Autodesk Inventor part; units mm, degrees
(part 2 of 2)
  arc A586 (72.5833, -71.3455) -> (69.8846, -69.0178) centre (57.5837, -86.0076) ccw projected
  arc A587 (72.1248, -72.4647) -> (72.5833, -71.3455) centre (0.3933, -42.4252) ccw projected
  arc A588 (68.5687, -72.23) -> (72.1248, -72.4647) centre (71.7232, -51.4931) ccw projected
  arc A589 (68.097, -73.2866) -> (68.5687, -72.23) centre (0.3933, -42.4252) ccw projected
  arc A590 (70.6457, -75.7776) -> (68.097, -73.2866) centre (54.7636, -89.4788) ccw projected
  arc A591 (70.1185, -76.8661) -> (70.6457, -75.7776) centre (0.3933, -42.4252) ccw projected
  arc A592 (66.5839, -76.4107) -> (70.1185, -76.8661) centre (71.0214, -55.9101) ccw projected
  arc A593 (66.0474, -77.436) -> (66.5839, -76.4107) centre (0.3933, -42.4252) ccw projected
  arc A594 (68.4363, -80.0806) -> (66.0474, -77.436) centre (51.7331, -92.768) ccw projected
  arc A595 (67.8425, -81.1342) -> (68.4363, -80.0806) centre (0.3933, -42.4252) ccw projected
  arc A596 (64.343, -80.4601) -> (67.8425, -81.1342) centre (70.0464, -60.275) ccw projected
  arc A597 (63.7437, -81.45) -> (64.343, -80.4601) centre (0.3933, -42.4252) ccw projected
  arc A598 (65.9637, -84.238) -> (63.7437, -81.45) centre (48.504, -95.8624) ccw projected
  arc A599 (65.3055, -85.2527) -> (65.9637, -84.238) centre (0.3933, -42.4252) ccw projected
  arc A600 (61.8547, -84.3622) -> (65.3055, -85.2527) centre (68.802, -64.5707) ccw projected
  arc A601 (61.195, -85.313) -> (61.8547, -84.3622) centre (0.3933, -42.4252) ccw projected
  arc A602 (63.2374, -88.2336) -> (61.195, -85.313) centre (45.0888, -98.7501) ccw projected
  arc A603 (62.5174, -89.2054) -> (63.2374, -88.2336) centre (0.3933, -42.4252) ccw projected
  arc A604 (59.1286, -88.1021) -> (62.5174, -89.2054) centre (67.2929, -68.7809) ccw projected
  arc A605 (58.4111, -89.01) -> (59.1286, -88.1021) centre (0.3933, -42.4252) ccw projected
  arc A606 (60.2679, -92.052) -> (58.4111, -89.01) centre (41.5006, -101.4198) ccw projected
  arc A607 (59.4889, -92.9771) -> (60.2679, -92.052) centre (0.3933, -42.4252) ccw projected
  arc A608 (56.1752, -91.6653) -> (59.4889, -92.9771) centre (65.525, -72.889) ccw projected
  arc A609 (55.4027, -92.5269) -> (56.1752, -91.6653) centre (0.3933, -42.4252) ccw projected
  arc A610 (57.0668, -95.6784) -> (55.4027, -92.5269) centre (37.7534, -103.8613) ccw projected
  arc A611 (56.2318, -96.5533) -> (57.0668, -95.6784) centre (0.3933, -42.4252) ccw projected
  arc A612 (53.0061, -95.038) -> (56.2318, -96.5533) centre (63.505, -76.8793) ccw projected
  arc A613 (52.1815, -95.8499) -> (53.0061, -95.038) centre (0.3933, -42.4252) ccw projected
  arc A614 (53.6464, -99.0987) -> (52.1815, -95.8499) centre (33.8617, -106.0651) ccw projected
  arc A615 (52.7586, -99.92) -> (53.6464, -99.0987) centre (0.3933, -42.4252) ccw projected
  arc A616 (49.6334, -98.2072) -> (52.7586, -99.92) centre (61.241, -80.7363) ccw projected
  arc A617 (48.7599, -98.9662) -> (49.6334, -98.2072) centre (0.3933, -42.4252) ccw projected
  arc A618 (50.0201, -102.2998) -> (48.7599, -98.9662) centre (29.8405, -108.0228) ccw projected
  arc A619 (49.0829, -103.0644) -> (50.0201, -102.2998) centre (0.3933, -42.4252) ccw projected
  arc A620 (46.0702, -101.1605) -> (49.0829, -103.0644) centre (58.7415, -84.445) ccw projected
  arc A621 (45.1512, -101.8637) -> (46.0702, -101.1605) centre (0.3933, -42.4252) ccw projected
  arc A622 (46.2017, -105.2693) -> (45.1512, -101.8637) centre (25.7053, -109.7266) ccw projected
  arc A623 (45.2188, -105.9741) -> (46.2017, -105.2693) centre (0.3933, -42.4252) ccw projected
  arc A624 (42.3303, -103.8866) -> (45.2188, -105.9741) centre (56.0162, -87.9912) ccw projected
  arc A625 (41.3694, -104.5313) -> (42.3303, -103.8866) centre (0.3933, -42.4252) ccw projected
  arc A626 (42.2061, -107.9956) -> (41.3694, -104.5313) centre (21.4723, -111.17) ccw projected
  arc A627 (41.1813, -108.6379) -> (42.2061, -107.9956) centre (0.3933, -42.4252) ccw projected
  arc A628 (38.4281, -106.3749) -> (41.1813, -108.6379) centre (53.0758, -91.3612) ccw projected
  arc A629 (37.429, -106.9587) -> (38.4281, -106.3749) centre (0.3933, -42.4252) ccw projected
  arc A630 (38.0487, -110.4682) -> (37.429, -106.9587) centre (17.1577, -112.3475) ccw projected
  arc A631 (36.986, -111.0456) -> (38.0487, -110.4682) centre (0.3933, -42.4252) ccw projected
  arc A632 (34.3788, -108.6158) -> (36.986, -111.0456) centre (49.9316, -94.5417) ccw projected
  arc A633 (33.3453, -109.1363) -> (34.3788, -108.6158) centre (0.3933, -42.4252) ccw projected
  arc A634 (33.7456, -112.6776) -> (33.3453, -109.1363) centre (12.7782, -113.2545) ccw projected
  arc A635 (32.6491, -113.1878) -> (33.7456, -112.6776) centre (0.3933, -42.4252) ccw projected
  arc A636 (30.198, -110.6006) -> (32.6491, -113.1878) centre (46.5957, -97.5207) ccw projected
  arc A637 (29.1342, -111.0559) -> (30.198, -110.6006) centre (0.3933, -42.4252) ccw projected
  arc A638 (29.3136, -114.6152) -> (29.1342, -111.0559) centre (8.3508, -113.8875) ccw projected
  arc A639 (28.1874, -115.0563) -> (29.3136, -114.6152) centre (0.3933, -42.4252) ccw projected
  arc A640 (25.902, -112.3217) -> (28.1874, -115.0563) centre (43.081, -100.2865) ccw projected
  arc A641 (24.8118, -112.71) -> (25.902, -112.3217) centre (0.3933, -42.4252) ccw projected
  arc A642 (24.7696, -116.2736) -> (24.8118, -112.71) centre (3.8926, -114.2439) ccw projected
  arc A643 (23.6182, -116.6437) -> (24.7696, -116.2736) centre (0.3933, -42.4252) ccw projected
  arc A644 (21.5072, -113.7724) -> (23.6182, -116.6437) centre (39.4013, -102.8285) ccw projected
  arc A645 (20.395, -114.0921) -> (21.5072, -113.7724) centre (0.3933, -42.4252) ccw projected
  arc A646 (20.1313, -117.6462) -> (20.395, -114.0921) centre (-0.5791, -114.3226) ccw projected
  arc A647 (18.9591, -117.944) -> (20.1313, -117.6462) centre (0.3933, -42.4252) ccw projected
  arc A648 (17.0307, -114.947) -> (18.9591, -117.944) centre (35.5705, -105.1367) ccw projected
  arc A649 (15.9008, -115.197) -> (17.0307, -114.947) centre (0.3933, -42.4252) ccw projected
  arc A650 (15.4167, -118.7278) -> (15.9008, -115.197) centre (-5.047, -114.123) ccw projected
  arc A651 (14.2282, -118.9522) -> (15.4167, -118.7278) centre (0.3933, -42.4252) ccw projected
  arc A652 (12.4899, -115.8411) -> (14.2282, -118.9522) centre (31.6037, -107.2024) ccw projected
  arc A653 (11.3466, -116.0203) -> (12.4899, -115.8411) centre (0.3933, -42.4252) ccw projected
  arc A654 (10.6439, -119.5142) -> (11.3466, -116.0203) centre (-9.494, -113.6461) ccw projected
  arc A655 (9.4438, -119.6643) -> (10.6439, -119.5142) centre (0.3933, -42.4252) ccw projected
  arc A656 (7.9022, -116.4511) -> (9.4438, -119.6643) centre (27.5162, -109.0174) ccw projected
  arc A657 (6.7501, -116.5589) -> (7.9022, -116.4511) centre (0.3933, -42.4252) ccw projected
  circle A658 centre (0.3933, -42.4252) radius 85.5443 projected
  circle A659 centre (0.3933, -42.4252) radius 82.55 projected
  circle A660 centre (0.3933, -42.4252) radius 81.28
  line L7 (-19.7673, 36.3148) -> (20.5539, 36.3148)
  line L8 (-77.8779, -20.5148) -> (-57.7172, 14.4044)
  line L9 (-57.7172, -99.2548) -> (-77.8779, -64.3356)
  line L10 (20.5539, -121.1652) -> (-19.7673, -121.1652)
  line L11 (78.6644, -64.3356) -> (58.5038, -99.2548)
  line L12 (58.5038, 14.4044) -> (78.6644, -20.5148)
  point P0 (0.3933, 36.3148)
  point P1 (-67.7976, -3.0552)
  point P2 (-67.7976, -81.7952)
  point P3 (0.3933, -121.1652)
  point P4 (68.5841, -81.7952)
  point P5 (68.5841, -3.0552)
  point P6 (78.6644, -20.5148)
  point P7 (58.5038, 14.4044)
  point P8 (-19.7673, -121.1652)
  dimension "d1" = 162.56
  dimension "d2" = 78.74
  dimension "d5" = 360
  constraints: 12 end point, 2 point on circle, 1 centre point, 1 coincident, 1 horizontal, 1 midpoint, 25 other
  measures "d1" diameter of A660
  measures "d2" distance of A660.centre point (0.393, 36.315)
extrude "Extrusion1" add sketch "Sketch2" along normal blind 7.62 contours A0 | L0 A1 | A101 A100 A248 A249 A99 A98 A250 A97 A96 A252 A95 A94 A253 A102 A93 A92 A91 A90 A89 A88 A87 A86 A85 A84 A83 A82 A81 A80 A79 A78 A77 A76 A75 A74 A73 A72 A71 A70 A69 A68 A67 A66 A65 A64 A63 A62 A61 A60 A59 A58 A57 A56 A55 A54 A53 A52 A51 A50 A49 A48 A47 A46 A45 A44 A43 A42 A41 A40 A39 A38 A37 A36 A35 A34 A33 A32 A31 A30 A29 A28 A27 A26 A25 A24 A23 A22 A21 A20 A19 A18 A17 A16 A15 A14 A13 A12 A11 A10 A9 A8 A7 A6 A5 A4 A3 A2 | A248 A247 A246 A245 A244 A243 A242 A241 A240 A239 A238 A237 A236 A235 A234 A233 A232 A231 A230 A229 A228 A227 A226 A225 A224 A223 A222 A221 A220 A219 A218 A217 A216 A215 A214 A213 A212 A211 A210 A209 A208 A207 A206 A205 A204 A203 A202 A201 A200 A199 A198 A197 A196 A195 A194 A193 A192 A191 A190 A189 A188 A187 A186 A185 A184 A183 A182 A181 A180 A179 A178 A177 A176 A175 A174 A173 A172 A171 A170 A169 A168 A167 A166 A165 A164 A163 A162 A161 A160 A159 A158 A157 A156 A155 A154 A153 A152 A151 A150 A149 A148 A147 A146 A145 A144 A143 A142 A141 A140 A139 A138 A137 A136 A135 A134 A133 A132 A131 A130 A129 A128 A127 A126 A125 A124 A123 A122 A121 A120 A119 A118 A117 A116 A115 A114 A113 A112 A111 A110 A109 A108 A107 A106 A105 A104 A103 A102 A94 A253 A252 A96 A251 A250 A98 A249 A100 | A100 A249 A248 | A249 A250 A98 A99 A100 | A98 A250 | A250 A251 A252 A96 A97 A98 | A96 A252 | A252 A253 A94 A95 A96 | A94 A102 A253 | L2 L3 L4 L5 L6 L1 | A255 A256 A257 A258 A259 A260 A261 A262 A263 A264 A265 A266 A267 A268 A269 A270 A271 A272 A273 A274 A275 A276 A277 A278 A279 A280 A281 A282 A283 A284 A285 A286 A287 A288 A289 A290 A291 A292 A293 A294 A295 A296 A297 A298 A299 A300 A301 A302 A303 A304 A305 A306 A307 A308 A309 A310 A311 A312 A313 A314 A315 A316 A317 A318 A319 A320 A321 A322 A323 A324 A325 A326 A327 A328 A329 A330 A331 A332 A333 A334 A335 A336 A337 A338 A339 A340 A341 A342 A343 A344 A345 A346 A347 A348 A349 A350 A351 A352 A353 A354 A355 A356 A357 A358 A359 A360 A361 A362 A363 A364 A365 A366 A367 A368 A369 A370 A371 A372 A373 A374 A375 A376 A377 A378 A379 A380 A381 A382 A383 A384 A385 A386 A387 A388 A389 A390 A391 A392 A393 A394 A395 A396 A397 A398 A399 A400 A401 A402 A403 A404 A405 A406 A407 A408 A409 A410 A411 A412 A413 A414 A415 A416 A417 A418 A419 A420 A421 A422 A423 A424 A425 A426 A427 A428 A429 A430 A431 A432 A433 A434 A435 A436 A437 A438 A439 A440 A441 A442 A443 A444 A445 A446 A447 A448 A449 A450 A451 A452 A453 A454 A455 A456 A457 A458 A459 A460 A461 A462 A463 A464 A465 A466 A467 A468 A469 A470 A471 A472 A473 A474 A475 A476 A477 A478 A479 A480 A481 A482 A483 A484 A485 A486 A487 A488 A489 A490 A491 A492 A493 A494 A495 A496 A497 A498 A499 A500 A501 A502 A503 A504 A505 A506 A507 A508 A509 A510 A511 A512 A513 A514 A515 A516 A517 A518 A519 A520 A521 A522 A523 A524 A525 A526 A527 A528 A529 A530 A531 A532 A533 A534 A535 A536 A537 A538 A539 A540 A541 A542 A543 A544 A545 A546 A547 A548 A549 A550 A551 A552 A553 A554 A555 A556 A557 A558 A559 A560 A561 A562 A563 A564 A565 A566 A567 A568 A569 A570 A571 A572 A573 A574 A575 A576 A577 A578 A579 A580 A581 A582 A583 A584 A585 A586 A587 A588 A589 A590 A591 A592 A593 A594 A595 A596 A597 A598 A599 A600 A601 A602 A603 A604 A605 A606 A607 A608 A609 A610 A611 A612 A613 A614 A615 A616 A617 A618 A619 A620 A621 A622 A623 A624 A625 A626 A627 A628 A629 A630 A631 A632 A633 A634 A635 A636 A637 A638 A639 A640 A641 A642 A643 A644 A645 A646 A647 A648 A649 A650 A651 A652 A653 A654 A655 A656 A657 A254 | A660 L11 L10 L9 L8 L7 L12
sketch "Sketch3" plane through (-0.3933, 42.4252, 8.89) normal (0, 0, 1) x (1, 0, 0)
  line L0 (3.5268, 9.2654) -> (-1.9537, 9.7195)
  line L1 (-1.9537, 9.7195) -> (-5.0872, 5.2004)
  line L2 (-5.0872, 5.2004) -> (-2.7402, 0.2271)
  line L3 (-2.7402, 0.2271) -> (2.7402, -0.2271)
  line L4 (2.7402, -0.2271) -> (5.8738, 4.2921)
  line L5 (5.8738, 4.2921) -> (3.5268, 9.2654)
  arc A0 (3.4869, -25.0828) -> (4.2324, -21.6038) centre (-12.0318, -19.9381) ccw
  arc A1 (2.2516, -25.1852) -> (3.4869, -25.0828) centre (0.3933, 4.7462) ccw
  arc A2 (0.9436, -21.8763) -> (2.2516, -25.1852) centre (16.7118, -17.5564) ccw
  arc A3 (-0.157, -21.8763) -> (0.9436, -21.8763) centre (0.3933, 4.7462) ccw
  arc A4 (-1.465, -25.1852) -> (-0.157, -21.8763) centre (-15.9252, -17.5564) ccw
  arc A5 (-2.7003, -25.0828) -> (-1.465, -25.1852) centre (0.3933, 4.7462) ccw
  arc A6 (-3.4458, -21.6038) -> (-2.7003, -25.0828) centre (12.8183, -19.9381) ccw
  arc A7 (-4.5315, -21.4226) -> (-3.4458, -21.6038) centre (0.3933, 4.7462) ccw
  arc A8 (-6.3662, -24.4711) -> (-4.5315, -21.4226) centre (-19.3735, -14.5662) ccw
  arc A9 (-7.5678, -24.1668) -> (-6.3662, -24.4711) centre (0.3933, 4.7462) ccw
  arc A10 (-7.7305, -20.6125) -> (-7.5678, -24.1668) centre (8.586, -21.6465) ccw
  arc A11 (-8.7715, -20.2551) -> (-7.7305, -20.6125) centre (0.3933, 4.7462) ccw
  arc A12 (-11.083, -22.9601) -> (-8.7715, -20.2551) centre (-22.2827, -11.0493) ccw
  arc A13 (-12.2182, -22.4621) -> (-11.083, -22.9601) centre (0.3933, 4.7462) ccw
  arc A14 (-11.7936, -18.9295) -> (-12.2182, -22.4621) centre (4.1301, -22.6351) ccw
  arc A15 (-12.7616, -18.4057) -> (-11.7936, -18.9295) centre (0.3933, 4.7462) ccw
  arc A16 (-15.4868, -20.6932) -> (-12.7616, -18.4057) centre (-24.5733, -7.1016) ccw
  arc A17 (-16.5245, -20.0153) -> (-15.4868, -20.6932) centre (0.3933, 4.7462) ccw
  arc A18 (-15.5243, -16.6007) -> (-16.5245, -20.0153) centre (-0.4277, -22.8767) ccw
  arc A19 (-16.3929, -15.9247) -> (-15.5243, -16.6007) centre (0.3933, 4.7462) ccw
  arc A20 (-19.4574, -17.7325) -> (-16.3929, -15.9247) centre (-26.1828, -2.8306) ccw
  arc A21 (-20.3694, -16.893) -> (-19.4574, -17.7325) centre (0.3933, 4.7462) ccw
  arc A22 (-18.8208, -13.6896) -> (-20.3694, -16.893) centre (-4.963, -22.3648) ccw
  arc A23 (-19.5663, -12.8798) -> (-18.8208, -13.6896) centre (0.3933, 4.7462) ccw
  arc A24 (-22.8866, -14.1586) -> (-19.5663, -12.8798) centre (-27.0675, 1.647) ccw
  arc A25 (-23.6479, -13.1804) -> (-22.8866, -14.1586) centre (0.3933, 4.7462) ccw
  arc A26 (-21.5932, -10.2756) -> (-23.6479, -13.1804) centre (-9.3523, -21.1134) ccw
  arc A27 (-22.1952, -9.3542) -> (-21.5932, -10.2756) centre (0.3933, 4.7462) ccw
  arc A28 (-25.6807, -10.069) -> (-22.1952, -9.3542) centre (-27.2031, 6.2092) ccw
  arc A29 (-26.2707, -8.9789) -> (-25.6807, -10.069) centre (0.3933, 4.7462) ccw
  arc A30 (-23.7659, -6.4519) -> (-26.2707, -8.9789) centre (-13.4758, -19.1567) ccw
  arc A31 (-24.208, -5.4439) -> (-23.7659, -6.4519) centre (0.3933, 4.7462) ccw
  arc A32 (-27.7636, -5.5753) -> (-24.208, -5.4439) centre (-26.5859, 10.7314) ccw
  arc A33 (-28.1661, -4.4029) -> (-27.7636, -5.5753) centre (0.3933, 4.7462) ccw
  arc A34 (-25.2795, -2.3227) -> (-28.1661, -4.4029) centre (-17.2209, -16.5479) ccw
  arc A35 (-25.5497, -1.2557) -> (-25.2795, -2.3227) centre (0.3933, 4.7462) ccw
  arc A36 (-29.0784, -0.8001) -> (-25.5497, -1.2557) centre (-25.2328, 15.0904) ccw
  arc A37 (-29.2825, 0.4226) -> (-29.0784, -0.8001) centre (0.3933, 4.7462) ccw
  arc A38 (-26.0929, 1.9993) -> (-29.2825, 0.4226) centre (-20.4856, -13.3583) ccw
  arc A39 (-26.1838, 3.0962) -> (-26.0929, 1.9993) centre (0.3933, 4.7462) ccw
  arc A40 (-29.5894, 4.1265) -> (-26.1838, 3.0962) centre (-23.1807, 19.1673) ccw
  arc A41 (-29.5894, 5.366) -> (-29.5894, 4.1265) centre (0.3933, 4.7462) ccw
  arc A42 (-26.1838, 6.3963) -> (-29.5894, 5.366) centre (-23.1807, -9.6748) ccw
  arc A43 (-26.0929, 7.4931) -> (-26.1838, 6.3963) centre (0.3933, 4.7462) ccw
  arc A44 (-29.2825, 9.0699) -> (-26.0929, 7.4931) centre (-20.4856, 22.8507) ccw
  arc A45 (-29.0784, 10.2925) -> (-29.2825, 9.0699) centre (0.3933, 4.7462) ccw
  arc A46 (-25.5497, 10.7482) -> (-29.0784, 10.2925) centre (-25.2328, -5.598) ccw
  arc A47 (-25.2795, 11.8152) -> (-25.5497, 10.7482) centre (0.3933, 4.7462) ccw
  arc A48 (-28.1661, 13.8954) -> (-25.2795, 11.8152) centre (-17.2209, 26.0404) ccw
  arc A49 (-27.7636, 15.0678) -> (-28.1661, 13.8954) centre (0.3933, 4.7462) ccw
  arc A50 (-24.208, 14.9364) -> (-27.7636, 15.0678) centre (-26.5859, -1.239) ccw
  arc A51 (-23.7659, 15.9444) -> (-24.208, 14.9364) centre (0.3933, 4.7462) ccw
  arc A52 (-26.2707, 18.4713) -> (-23.7659, 15.9444) centre (-13.4758, 28.6491) ccw
  arc A53 (-25.6807, 19.5615) -> (-26.2707, 18.4713) centre (0.3933, 4.7462) ccw
  arc A54 (-22.1952, 18.8467) -> (-25.6807, 19.5615) centre (-27.2031, 3.2833) ccw
  arc A55 (-21.5932, 19.7681) -> (-22.1952, 18.8467) centre (0.3933, 4.7462) ccw
  arc A56 (-23.6479, 22.6729) -> (-21.5932, 19.7681) centre (-9.3523, 30.6059) ccw
  arc A57 (-22.8866, 23.6511) -> (-23.6479, 22.6729) centre (0.3933, 4.7462) ccw
  arc A58 (-19.5663, 22.3723) -> (-22.8866, 23.6511) centre (-27.0675, 7.8455) ccw
  arc A59 (-18.8208, 23.1821) -> (-19.5663, 22.3723) centre (0.3933, 4.7462) ccw
  arc A60 (-20.3694, 26.3854) -> (-18.8208, 23.1821) centre (-4.963, 31.8573) ccw
  arc A61 (-19.4574, 27.225) -> (-20.3694, 26.3854) centre (0.3933, 4.7462) ccw
  arc A62 (-16.3929, 25.4171) -> (-19.4574, 27.225) centre (-26.1828, 12.3231) ccw
  arc A63 (-15.5243, 26.0932) -> (-16.3929, 25.4171) centre (0.3933, 4.7462) ccw
  arc A64 (-16.5245, 29.5077) -> (-15.5243, 26.0932) centre (-0.4277, 32.3691) ccw
  arc A65 (-15.4868, 30.1857) -> (-16.5245, 29.5077) centre (0.3933, 4.7462) ccw
  arc A66 (-12.7616, 27.8981) -> (-15.4868, 30.1857) centre (-24.5733, 16.594) ccw
  arc A67 (-11.7936, 28.422) -> (-12.7616, 27.8981) centre (0.3933, 4.7462) ccw
  arc A68 (-12.2182, 31.9546) -> (-11.7936, 28.422) centre (4.1301, 32.1275) ccw
  arc A69 (-11.083, 32.4525) -> (-12.2182, 31.9546) centre (0.3933, 4.7462) ccw
  arc A70 (-8.7715, 29.7476) -> (-11.083, 32.4525) centre (-22.2827, 20.5418) ccw
  arc A71 (-7.7305, 30.105) -> (-8.7715, 29.7476) centre (0.3933, 4.7462) ccw
  arc A72 (-7.5678, 33.6593) -> (-7.7305, 30.105) centre (8.586, 31.139) ccw
  arc A73 (-6.3662, 33.9636) -> (-7.5678, 33.6593) centre (0.3933, 4.7462) ccw
  arc A74 (-4.5315, 30.9151) -> (-6.3662, 33.9636) centre (-19.3735, 24.0587) ccw
  arc A75 (-3.4458, 31.0962) -> (-4.5315, 30.9151) centre (0.3933, 4.7462) ccw
  arc A76 (-2.7003, 34.5753) -> (-3.4458, 31.0962) centre (12.8183, 29.4306) ccw
  arc A77 (-1.465, 34.6777) -> (-2.7003, 34.5753) centre (0.3933, 4.7462) ccw
  arc A78 (-0.157, 31.3688) -> (-1.465, 34.6777) centre (-15.9252, 27.0488) ccw
  arc A79 (0.9436, 31.3688) -> (-0.157, 31.3688) centre (0.3933, 4.7462) ccw
  arc A80 (2.2516, 34.6777) -> (0.9436, 31.3688) centre (16.7118, 27.0488) ccw
  arc A81 (3.4869, 34.5753) -> (2.2516, 34.6777) centre (0.3933, 4.7462) ccw
  arc A82 (4.2324, 31.0962) -> (3.4869, 34.5753) centre (-12.0318, 29.4306) ccw
  arc A83 (5.318, 30.9151) -> (4.2324, 31.0962) centre (0.3933, 4.7462) ccw
  arc A84 (7.1528, 33.9636) -> (5.318, 30.9151) centre (20.1601, 24.0587) ccw
  arc A85 (8.3544, 33.6593) -> (7.1528, 33.9636) centre (0.3933, 4.7462) ccw
  arc A86 (8.5171, 30.105) -> (8.3544, 33.6593) centre (-7.7994, 31.139) ccw
  arc A87 (9.5581, 29.7476) -> (8.5171, 30.105) centre (0.3933, 4.7462) ccw
  arc A88 (11.8696, 32.4525) -> (9.5581, 29.7476) centre (23.0692, 20.5418) ccw
  arc A89 (13.0048, 31.9546) -> (11.8696, 32.4525) centre (0.3933, 4.7462) ccw
  arc A90 (12.5802, 28.422) -> (13.0048, 31.9546) centre (-3.3436, 32.1275) ccw
  arc A91 (13.5482, 27.8981) -> (12.5802, 28.422) centre (0.3933, 4.7462) ccw
  arc A92 (16.2734, 30.1857) -> (13.5482, 27.8981) centre (25.3598, 16.594) ccw
  arc A93 (17.3111, 29.5077) -> (16.2734, 30.1857) centre (0.3933, 4.7462) ccw
  arc A94 (16.3109, 26.0932) -> (17.3111, 29.5077) centre (1.2142, 32.3691) ccw
  arc A95 (17.1795, 25.4171) -> (16.3109, 26.0932) centre (0.3933, 4.7462) ccw
  arc A96 (20.244, 27.225) -> (17.1795, 25.4171) centre (26.9694, 12.3231) ccw
  arc A97 (21.156, 26.3854) -> (20.244, 27.225) centre (0.3933, 4.7462) ccw
  arc A98 (19.6074, 23.1821) -> (21.156, 26.3854) centre (5.7496, 31.8573) ccw
  arc A99 (20.3528, 22.3723) -> (19.6074, 23.1821) centre (0.3933, 4.7462) ccw
  arc A100 (23.6731, 23.6511) -> (20.3528, 22.3723) centre (27.854, 7.8455) ccw
  arc A101 (24.4345, 22.6729) -> (23.6731, 23.6511) centre (0.3933, 4.7462) ccw
  arc A102 (22.3798, 19.7681) -> (24.4345, 22.6729) centre (10.1389, 30.6059) ccw
  arc A103 (22.9818, 18.8467) -> (22.3798, 19.7681) centre (0.3933, 4.7462) ccw
  arc A104 (26.4673, 19.5615) -> (22.9818, 18.8467) centre (27.9896, 3.2833) ccw
  arc A105 (27.0572, 18.4713) -> (26.4673, 19.5615) centre (0.3933, 4.7462) ccw
  arc A106 (24.5524, 15.9444) -> (27.0572, 18.4713) centre (14.2623, 28.6491) ccw
  arc A107 (24.9945, 14.9364) -> (24.5524, 15.9444) centre (0.3933, 4.7462) ccw
  arc A108 (28.5502, 15.0678) -> (24.9945, 14.9364) centre (27.3725, -1.239) ccw
  arc A109 (28.9527, 13.8954) -> (28.5502, 15.0678) centre (0.3933, 4.7462) ccw
  arc A110 (26.0661, 11.8152) -> (28.9527, 13.8954) centre (18.0075, 26.0404) ccw
  arc A111 (26.3363, 10.7482) -> (26.0661, 11.8152) centre (0.3933, 4.7462) ccw
  arc A112 (29.865, 10.2925) -> (26.3363, 10.7482) centre (26.0194, -5.598) ccw
  arc A113 (30.069, 9.0699) -> (29.865, 10.2925) centre (0.3933, 4.7462) ccw
  arc A114 (26.8794, 7.4931) -> (30.069, 9.0699) centre (21.2721, 22.8507) ccw
  arc A115 (26.9703, 6.3963) -> (26.8794, 7.4931) centre (0.3933, 4.7462) ccw
  arc A116 (30.376, 5.366) -> (26.9703, 6.3963) centre (23.9673, -9.6748) ccw
  arc A117 (30.376, 4.1265) -> (30.376, 5.366) centre (0.3933, 4.7462) ccw
  arc A118 (26.9703, 3.0962) -> (30.376, 4.1265) centre (23.9673, 19.1673) ccw
  arc A119 (26.8794, 1.9993) -> (26.9703, 3.0962) centre (0.3933, 4.7462) ccw
  arc A120 (30.069, 0.4226) -> (26.8794, 1.9993) centre (21.2721, -13.3583) ccw
  arc A121 (29.865, -0.8001) -> (30.069, 0.4226) centre (0.3933, 4.7462) ccw
  arc A122 (26.3363, -1.2557) -> (29.865, -0.8001) centre (26.0194, 15.0904) ccw
  arc A123 (26.0661, -2.3227) -> (26.3363, -1.2557) centre (0.3933, 4.7462) ccw
  arc A124 (28.9527, -4.4029) -> (26.0661, -2.3227) centre (18.0075, -16.5479) ccw
  arc A125 (28.5502, -5.5753) -> (28.9527, -4.4029) centre (0.3933, 4.7462) ccw
  arc A126 (24.9945, -5.4439) -> (28.5502, -5.5753) centre (27.3725, 10.7314) ccw
  arc A127 (24.5524, -6.4519) -> (24.9945, -5.4439) centre (0.3933, 4.7462) ccw
  arc A128 (27.0572, -8.9789) -> (24.5524, -6.4519) centre (14.2623, -19.1567) ccw
  arc A129 (26.4673, -10.069) -> (27.0572, -8.9789) centre (0.3933, 4.7462) ccw
  arc A130 (22.9818, -9.3542) -> (26.4673, -10.069) centre (27.9896, 6.2092) ccw
  arc A131 (22.3798, -10.2756) -> (22.9818, -9.3542) centre (0.3933, 4.7462) ccw
  arc A132 (24.4345, -13.1804) -> (22.3798, -10.2756) centre (10.1389, -21.1134) ccw
  arc A133 (23.6731, -14.1586) -> (24.4345, -13.1804) centre (0.3933, 4.7462) ccw
  arc A134 (20.3528, -12.8798) -> (23.6731, -14.1586) centre (27.854, 1.647) ccw
  arc A135 (19.6074, -13.6896) -> (20.3528, -12.8798) centre (0.3933, 4.7462) ccw
  arc A136 (21.156, -16.893) -> (19.6074, -13.6896) centre (5.7496, -22.3648) ccw
  arc A137 (20.244, -17.7325) -> (21.156, -16.893) centre (0.3933, 4.7462) ccw
  arc A138 (17.1795, -15.9247) -> (20.244, -17.7325) centre (26.9694, -2.8306) ccw
  arc A139 (16.3109, -16.6007) -> (17.1795, -15.9247) centre (0.3933, 4.7462) ccw
  arc A140 (17.3111, -20.0153) -> (16.3109, -16.6007) centre (1.2142, -22.8767) ccw
  arc A141 (16.2734, -20.6932) -> (17.3111, -20.0153) centre (0.3933, 4.7462) ccw
  arc A142 (13.5482, -18.4057) -> (16.2734, -20.6932) centre (25.3598, -7.1016) ccw
  arc A143 (12.5802, -18.9295) -> (13.5482, -18.4057) centre (0.3933, 4.7462) ccw
  arc A144 (13.0048, -22.4621) -> (12.5802, -18.9295) centre (-3.3436, -22.6351) ccw
  arc A145 (11.8696, -22.9601) -> (13.0048, -22.4621) centre (0.3933, 4.7462) ccw
  arc A146 (9.5581, -20.2551) -> (11.8696, -22.9601) centre (23.0692, -11.0493) ccw
  arc A147 (8.5171, -20.6125) -> (9.5581, -20.2551) centre (0.3933, 4.7462) ccw
  arc A148 (8.3544, -24.1668) -> (8.5171, -20.6125) centre (-7.7994, -21.6465) ccw
  arc A149 (7.1528, -24.4711) -> (8.3544, -24.1668) centre (0.3933, 4.7462) ccw
  arc A150 (5.318, -21.4226) -> (7.1528, -24.4711) centre (20.1601, -14.5662) ccw
  arc A151 (4.2324, -21.6038) -> (5.318, -21.4226) centre (0.3933, 4.7462) ccw
  circle A152 centre (0.3933, 4.7462) radius 14.605
  point P0 (0.3933, -42.4252)
extrude "Extrusion2" cut sketch "Sketch3" against normal through all contours L5 L4 L3 L2 L1 L0 | A152
chamfer "Chamfer1" distance 1 angle 45 1 edges at (-14.605, 47.1714, 8.89)
pattern_circular "Circular Pattern1" count 3 over 360 about axis through (0, 0, 1.27) along (0, 0, 1) of "Extrusion2", "Chamfer1"
sketch "Sketch4" plane through (-0.3933, 42.4252, 8.89) normal (0, 0, 1) x (1, 0, 0)
  arc A0 (0.495, -45.4235) -> (0.2916, -45.4235) centre (0.3933, -42.4252) ccw projected
  line L0 (0.2916, -45.4235) -> (0.495, -45.4235) projected
  arc A1 (-5.2339, -23.0564) -> (-5.3005, -26.6101) centre (8.4164, -25.0898) ccw projected
  arc A2 (-5.3005, -26.6101) -> (-6.2823, -26.9988) centre (0.3933, -42.4252) ccw projected
  arc A3 (-6.2823, -26.9988) -> (-8.7636, -24.4539) centre (-17.3222, -35.2804) ccw projected
  arc A4 (-8.7636, -24.4539) -> (-9.8739, -25.0643) centre (0.3933, -42.4252) ccw projected
  arc A5 (-9.8739, -25.0643) -> (-9.0547, -28.5229) centre (3.8531, -23.6391) ccw projected
  arc A6 (-9.0547, -28.5229) -> (-9.909, -29.1436) centre (0.3933, -42.4252) ccw projected
  arc A7 (-9.909, -29.1436) -> (-12.9452, -27.2957) centre (-18.5425, -39.9105) ccw projected
  arc A8 (-12.9452, -27.2957) -> (-13.8688, -28.1631) centre (0.3933, -42.4252) ccw projected
  arc A9 (-13.8688, -28.1631) -> (-12.2152, -31.3093) centre (-0.9275, -23.3689) ccw projected
  arc A10 (-12.2152, -31.3093) -> (-12.8883, -32.1229) centre (0.3933, -42.4252) ccw projected
  arc A11 (-12.8883, -32.1229) -> (-16.2887, -31.0882) centre (-18.5729, -44.6986) ccw projected
  arc A12 (-16.2887, -31.0882) -> (-16.9676, -32.158) centre (0.3933, -42.4252) ccw projected
  arc A13 (-16.9676, -32.158) -> (-14.5835, -34.7941) centre (-5.6251, -24.296) ccw projected
  arc A14 (-14.5835, -34.7941) -> (-15.0331, -35.7496) centre (0.3933, -42.4252) ccw projected
  arc A15 (-15.0331, -35.7496) -> (-18.584, -35.593) centre (-17.4117, -49.3439) ccw projected
  arc A16 (-18.584, -35.593) -> (-18.9755, -36.798) centre (0.3933, -42.4252) ccw projected
  arc A17 (-18.9755, -36.798) -> (-16.0107, -38.7585) centre (-9.9445, -26.3623) ccw projected
  arc A18 (-16.0107, -38.7585) -> (-16.2086, -39.7957) centre (0.3933, -42.4252) ccw projected
  arc A19 (-16.2086, -39.7957) -> (-19.6869, -40.5271) centre (-15.1317, -53.5545) ccw projected
  arc A20 (-19.6869, -40.5271) -> (-19.7664, -41.7916) centre (0.3933, -42.4252) ccw projected
  arc A21 (-19.7664, -41.7916) -> (-16.4072, -42.9532) centre (-13.6144, -29.4379) ccw projected
  arc A22 (-16.4072, -42.9532) -> (-16.3409, -44.007) centre (0.3933, -42.4252) ccw projected
  arc A23 (-16.3409, -44.007) -> (-19.5281, -45.5804) centre (-11.8762, -57.0657) ccw projected
  arc A24 (-19.5281, -45.5804) -> (-19.2906, -46.8251) centre (0.3933, -42.4252) ccw projected
  arc A25 (-19.2906, -46.8251) -> (-15.7481, -47.1147) centre (-16.4042, -33.3295) ccw projected
  arc A26 (-15.7481, -47.1147) -> (-15.4218, -48.119) centre (0.3933, -42.4252) ccw projected
  arc A27 (-15.4218, -48.119) -> (-18.1175, -50.4355) centre (-7.8498, -59.6571) ccw projected
  arc A28 (-18.1175, -50.4355) -> (-17.578, -51.582) centre (0.3933, -42.4252) ccw projected
  arc A29 (-17.578, -51.582) -> (-14.0748, -50.9816) centre (-18.1385, -37.7926) ccw projected
  arc A30 (-14.0748, -50.9816) -> (-13.509, -51.8732) centre (0.3933, -42.4252) ccw projected
  arc A31 (-13.509, -51.8732) -> (-15.5439, -54.7873) centre (-3.3054, -61.1657) ccw projected
  arc A32 (-15.5439, -54.7873) -> (-14.7362, -55.7636) centre (0.3933, -42.4252) ccw projected
  arc A33 (-14.7362, -55.7636) -> (-11.4923, -54.3108) centre (-18.7083, -42.5468) ccw projected
  arc A34 (-11.4923, -54.3108) -> (-10.7226, -55.0337) centre (0.3933, -42.4252) ccw projected
  arc A35 (-10.7226, -55.0337) -> (-11.9689, -58.3624) centre (1.4713, -61.4968) ccw projected
  arc A36 (-11.9689, -58.3624) -> (-10.9438, -59.1071) centre (0.3933, -42.4252) ccw projected
  arc A37 (-10.9438, -59.1071) -> (-8.1631, -56.8933) centre (-18.078, -47.2933) ccw projected
  arc A38 (-8.1631, -56.8933) -> (-7.2378, -57.402) centre (0.3933, -42.4252) ccw projected
  arc A39 (-7.2378, -57.402) -> (-7.6171, -60.936) centre (6.1804, -60.6295) ccw projected
  arc A40 (-7.6171, -60.936) -> (-6.439, -61.4025) centre (0.3933, -42.4252) ccw projected
  arc A41 (-6.439, -61.4025) -> (-4.2962, -58.5666) centre (-16.287, -51.734) ccw projected
  arc A42 (-4.2962, -58.5666) -> (-3.2734, -58.8292) centre (0.3933, -42.4252) ccw projected
  arc A43 (-3.2734, -58.8292) -> (-2.7619, -62.3466) centre (10.5258, -58.6184) ccw projected
  arc A44 (-2.7619, -62.3466) -> (-1.5049, -62.5054) centre (0.3933, -42.4252) ccw projected
  arc A45 (-1.5049, -62.5054) -> (-0.1347, -59.2257) centre (-13.448, -55.5898) ccw projected
  arc A46 (-0.1347, -59.2257) -> (0.9213, -59.2257) centre (0.3933, -42.4252) ccw projected
  arc A47 (0.9213, -59.2257) -> (2.2914, -62.5054) centre (14.2345, -55.5898) ccw projected
  arc A48 (2.2914, -62.5054) -> (3.5485, -62.3466) centre (0.3933, -42.4252) ccw projected
  arc A49 (3.5485, -62.3466) -> (4.06, -58.8292) centre (-9.7392, -58.6184) ccw projected
  arc A50 (4.06, -58.8292) -> (5.0828, -58.5666) centre (0.3933, -42.4252) ccw projected
  arc A51 (5.0828, -58.5666) -> (7.2255, -61.4025) centre (17.0736, -51.734) ccw projected
  arc A52 (7.2255, -61.4025) -> (8.4036, -60.936) centre (0.3933, -42.4252) ccw projected
  arc A53 (8.4036, -60.936) -> (8.0243, -57.402) centre (-5.3938, -60.6295) ccw projected
  arc A54 (8.0243, -57.402) -> (8.9497, -56.8933) centre (0.3933, -42.4252) ccw projected
  arc A55 (8.9497, -56.8933) -> (11.7303, -59.1071) centre (18.8646, -47.2933) ccw projected
  arc A56 (11.7303, -59.1071) -> (12.7554, -58.3624) centre (0.3933, -42.4252) ccw projected
  arc A57 (12.7554, -58.3624) -> (11.5092, -55.0337) centre (-0.6848, -61.4968) ccw projected
  arc A58 (11.5092, -55.0337) -> (12.2789, -54.3108) centre (0.3933, -42.4252) ccw projected
  arc A59 (12.2789, -54.3108) -> (15.5228, -55.7636) centre (19.4949, -42.5468) ccw projected
  arc A60 (15.5228, -55.7636) -> (16.3305, -54.7873) centre (0.3933, -42.4252) ccw projected
  arc A61 (16.3305, -54.7873) -> (14.2955, -51.8732) centre (4.092, -61.1657) ccw projected
  arc A62 (14.2955, -51.8732) -> (14.8613, -50.9816) centre (0.3933, -42.4252) ccw projected
  arc A63 (14.8613, -50.9816) -> (18.3646, -51.582) centre (18.925, -37.7926) ccw projected
  arc A64 (18.3646, -51.582) -> (18.9041, -50.4355) centre (0.3933, -42.4252) ccw projected
  arc A65 (18.9041, -50.4355) -> (16.2084, -48.119) centre (8.6364, -59.6571) ccw projected
  arc A66 (16.2084, -48.119) -> (16.5347, -47.1147) centre (0.3933, -42.4252) ccw projected
  arc A67 (16.5347, -47.1147) -> (20.0772, -46.8251) centre (17.1907, -33.3295) ccw projected
  arc A68 (20.0772, -46.8251) -> (20.3146, -45.5804) centre (0.3933, -42.4252) ccw projected
  arc A69 (20.3146, -45.5804) -> (17.1275, -44.007) centre (12.6628, -57.0657) ccw projected
  arc A70 (17.1275, -44.007) -> (17.1938, -42.9532) centre (0.3933, -42.4252) ccw projected
  arc A71 (17.1938, -42.9532) -> (20.553, -41.7916) centre (14.401, -29.4379) ccw projected
  arc A72 (20.553, -41.7916) -> (20.4735, -40.5271) centre (0.3933, -42.4252) ccw projected
  arc A73 (20.4735, -40.5271) -> (16.9952, -39.7957) centre (15.9183, -53.5545) ccw projected
  arc A74 (16.9952, -39.7957) -> (16.7973, -38.7585) centre (0.3933, -42.4252) ccw projected
  arc A75 (16.7973, -38.7585) -> (19.7621, -36.798) centre (10.7311, -26.3623) ccw projected
  arc A76 (19.7621, -36.798) -> (19.3706, -35.593) centre (0.3933, -42.4252) ccw projected
  arc A77 (19.3706, -35.593) -> (15.8197, -35.7496) centre (18.1983, -49.3439) ccw projected
  arc A78 (15.8197, -35.7496) -> (15.3701, -34.7941) centre (0.3933, -42.4252) ccw projected
  arc A79 (15.3701, -34.7941) -> (17.7542, -32.158) centre (6.4116, -24.296) ccw projected
  arc A80 (17.7542, -32.158) -> (17.0752, -31.0882) centre (0.3933, -42.4252) ccw projected
  arc A81 (17.0752, -31.0882) -> (13.6749, -32.1229) centre (19.3595, -44.6986) ccw projected
  arc A82 (13.6749, -32.1229) -> (13.0018, -31.3093) centre (0.3933, -42.4252) ccw projected
  arc A83 (13.0018, -31.3093) -> (14.6554, -28.1631) centre (1.714, -23.3689) ccw projected
  arc A84 (14.6554, -28.1631) -> (13.7317, -27.2957) centre (0.3933, -42.4252) ccw projected
  arc A85 (13.7317, -27.2957) -> (10.6955, -29.1436) centre (19.329, -39.9105) ccw projected
  arc A86 (10.6955, -29.1436) -> (9.8412, -28.5229) centre (0.3933, -42.4252) ccw projected
  arc A87 (9.8412, -28.5229) -> (10.6605, -25.0643) centre (-3.0666, -23.6391) ccw projected
  arc A88 (10.6605, -25.0643) -> (9.5501, -24.4539) centre (0.3933, -42.4252) ccw projected
  arc A89 (9.5501, -24.4539) -> (7.0689, -26.9988) centre (18.1088, -35.2804) ccw projected
  arc A90 (7.0689, -26.9988) -> (6.0871, -26.6101) centre (0.3933, -42.4252) ccw projected
  arc A91 (6.0871, -26.6101) -> (6.0204, -23.0564) centre (-7.6298, -25.0898) ccw projected
  arc A92 (6.0204, -23.0564) -> (4.7932, -22.7413) centre (0.3933, -42.4252) ccw projected
  arc A93 (4.7932, -22.7413) -> (3.0228, -25.8233) centre (15.7754, -31.0992) ccw projected
  arc A94 (3.0228, -25.8233) -> (1.9751, -25.691) centre (0.3933, -42.4252) ccw projected
  arc A95 (1.9751, -25.691) -> (1.0268, -22.2655) centre (-11.6889, -27.6297) ccw projected
  arc A96 (1.0268, -22.2655) -> (-0.2403, -22.2655) centre (0.3933, -42.4252) ccw projected
  arc A97 (-0.2403, -22.2655) -> (-1.1886, -25.691) centre (12.4754, -27.6297) ccw projected
  arc A98 (-1.1886, -25.691) -> (-2.2362, -25.8233) centre (0.3933, -42.4252) ccw projected
  arc A99 (-2.2362, -25.8233) -> (-4.0066, -22.7413) centre (-14.9888, -31.0992) ccw projected
  arc A100 (-4.0066, -22.7413) -> (-5.2339, -23.0564) centre (0.3933, -42.4252) ccw projected
  arc A101 (1.0086, -44.8483) -> (-0.222, -44.8483) centre (0.3933, -42.4252) ccw projected
  line L1 (-15.1067, -57.9252) -> (15.8933, -57.9252) construction
  line L2 (15.8933, -57.9252) -> (15.8933, -26.9252) construction
  line L3 (15.8933, -26.9252) -> (-15.1067, -26.9252) construction
  line L4 (-15.1067, -26.9252) -> (-15.1067, -57.9252) construction
  line L5 (-15.1067, -57.9252) -> (15.8933, -26.9252) construction
  line L6 (15.8933, -57.9252) -> (-15.1067, -26.9252) construction
  circle A102 centre (-15.1067, -26.9252) radius 3.175
  circle A103 centre (15.8933, -26.9252) radius 3.175
  circle A104 centre (15.8933, -57.9252) radius 3.175
  circle A105 centre (-15.1067, -57.9252) radius 3.175
  point P0 (0.3933, -42.4252)
  point P1 (14.1509, -55.271)
  point P2 (12.7402, -58.298)
  point P3 (12.7492, -58.3672)
  point P4 (16.3266, -54.7799)
  point P5 (-15.54, -54.7799)
  point P6 (-11.9626, -58.3672)
  point P7 (-11.9537, -58.298)
  point P8 (-13.3644, -55.271)
  dimension "d18" = 31
  dimension "d19" = 31
  dimension "d20" = 6.35
  dimension "d21" = 6.35
  dimension "d22" = 6.35
  dimension "d23" = 6.35
  constraints: 12 end point, 4 centre point, 4 coincident, 2 midpoint, 2 parallel, 1 horizontal, 1 perpendicular
  measures "d18" distance of L3.end L2.end
  measures "d19" distance of L2.end L1.end
  measures "d20" diameter of A102
  measures "d21" diameter of A103
  measures "d22" diameter of A104
  measures "d23" diameter of A105
extrude "Extrusion3" add sketch "Sketch4" along normal blind 10.16 contours A102 A9 A8 A7 | A7 A8 A9 A102 | A103 A83 A84 A85 | A85 A84 A83 A103 | A105 A33 A32 A31 | A31 A32 A33 A105 A35 A36 | A36 A35 A105 | A104 A56 A57 A59 A60 A61 | A61 A60 A59 A104 | A104 A57 A56
sketch "Sketch6" plane through (-0.3933, 42.4252, 1.27) normal (0, 0, -1) x (-1, 0, 0)
  circle A0 centre (15.1067, -57.9252) radius 3.175 projected
  circle A1 centre (15.1067, -26.9252) radius 3.175 projected
  circle A2 centre (-15.8933, -26.9252) radius 3.175 projected
  circle A3 centre (-15.8933, -57.9252) radius 3.175 projected
  point P0 (-0.3933, -42.4252)
hole "Hole2" at (-15.5, -15.5, 1.27) at (-15.5, 15.5, 1.27) at (15.5, -15.5, 1.27) at (15.5, 15.5, 1.27) direction (0, 0, 1) diameter 3.5 end through all counterbore diameter 6.35 counterbore depth 4.7625
chamfer "Chamfer2" distance 2 angle 45 4 edges at (-18.6441, -15.058, 8.89) (-18.675, 15.5, 8.89) (15.0667, -18.6453, 8.89) (12.325, 15.5, 8.89)
chamfer "Chamfer3" distance 0.4 angle 45 4 edges at (-15.5, -17.25, 19.05) (-15.5, 13.75, 19.05) (15.5, 13.75, 19.05) (15.5, -17.25, 19.05)
sketch "Sketch7" plane through (-0.3933, 42.4252, 8.89) normal (0, 0, 1) x (1, 0, 0)
  arc A0 (78.6644, -64.3356) -> (78.6644, -20.5148) centre (0.3933, -42.4252) ccw projected
  point P0 (0.3933, -42.4252)
  constraints: 1 coincident
hole "Hole3" at (0, 0, 8.89) direction (0, 0, -1) diameter 6.5 end through all countersink diameter 9.525 countersink angle 82
sketch "Sketch9" plane through (58.1105, 56.8296, 8.89) normal (0.8660254, 0.5, 0) x (0, 0, -1)
  line L0 (8.8265, -105.7049) -> (8.8265, 65.3836) projected
  circle A0 centre (6.3265, -8.89) radius 2.5
  line L1 (7.62, -40.3212) -> (7.62, 0) projected
  line L2 (7.62, 0) -> (0, 0) projected
  line L3 (0, -40.3212) -> (0, 0) projected
  line L4 (7.62, -40.3212) -> (0, -40.3212) projected
  line L5 (7.62, 0) -> (0, 0) projected
  point P0 (8.89, -20.1606)
  dimension "d55" = 5
  dimension "d81" = 8.89
  constraints: 1 centre point, 1 tangent
  measures "d55" diameter of A0
  measures "d81" distance from line of L2 A0.centre
hole "Hole4" at (62.5555, 49.1306, 2.5635) direction (-0.8660254, -0.5, 0) diameter 6 depth 6.35
sketch "Sketch10" plane through (57.0563, 45.9556, 2.5635) normal (0.8660254, 0.5, 0) x (0, 0, -1)
  arc A0 (1.2935, 2.7068) -> (1.2935, -2.7068) centre (0, 0) ccw projected
  point P0 (2.5635, -11.2706)
  point P1 (0, 0)
  constraints: 1 coincident
hole "Hole5" at (57.0563, 45.9556, 2.5635) direction (-0.8660254, -0.5, 0) diameter 5 depth 6
sketch "Sketch11" plane through (51.8601, 42.9556, 2.5635) normal (0.8660254, 0.5, 0) x (0, 0, -1)
  arc A0 (1.2935, 2.1394) -> (1.2935, -2.1394) centre (0, 0) ccw projected
  point P0 (2.5635, -11.2706)
  constraints: 1 coincident
hole "Hole6" at (51.8601, 42.9556, 2.5635) direction (-0.8660254, -0.5, 0) diameter 4 depth 6
sketch "Sketch12" plane through (58.1105, 56.8296, 8.89) normal (0.8660254, 0.5, 0) x (0, 0, -1)
  line L0 (7.62, 0) -> (7.62, -40.3212) projected
  line L1 (7.62, -20.1606) -> (0, -20.1606)
  line L2 (0, -40.3212) -> (0, 0) projected
  point P0 (8.89, -20.1606)
  constraints: 2 end point, 2 midpoint
ref_plane "Work Plane2" through (68.1908, 39.37, 1.27) normal (-0.5, 0.8660254, 0) x (0, 0, 1)
sketch "Sketch14" plane through (57.0563, 45.9556, 2.5635) normal (0.8660254, 0.5, 0) x (0, 0, -1)
  arc A0 (1.2935, 1.5254) -> (1.2935, -1.5254) centre (0, 0) ccw projected
  line L0 (1.2935, 2.1394) -> (1.2935, 1.5254) projected
  arc A1 (1.2935, 2.1394) -> (1.2935, -2.1394) centre (0, 0) ccw projected
  line L1 (1.2935, -1.5254) -> (1.2935, -2.1394) projected
  arc A2 (1.2935, 2.1394) -> (1.2935, -2.1394) centre (0, 0) ccw projected
  line L2 (1.2935, 2.7068) -> (1.2935, 2.1394) projected
  arc A3 (1.2935, 2.7068) -> (1.2935, -2.7068) centre (0, 0) ccw projected
  line L3 (1.2935, -2.1394) -> (1.2935, -2.7068) projected
  line L4 (1.2935, -1.5254) -> (1.2935, 1.5254)
  point P0 (2.5635, -11.2706)
  point P1 (1.2935, 2.1394)
  point P2 (1.2935, -2.1394)
  constraints: 2 end point, 1 vertical
extrude "Extrusion5" add sketch "Sketch14" along normal blind 2.3813 contours A0 L1 A1 L0 | A1 L3 A3 L2
sketch "Sketch15" plane through (-0.3933, 42.4252, 1.27) normal (0, 0, -1) x (-1, 0, 0)
  line L0 (-53.5034, -1.6346) -> (-58.6996, 1.3654) projected
  line L1 (-51.0034, 2.6955) -> (-56.1996, 5.6955) projected
  line L2 (-58.6996, 1.3654) -> (-56.1996, 5.6955) projected
  line L3 (-51.0034, 2.6955) -> (-53.5034, -1.6346) projected
  point P0 (-0.3933, -42.4252)
  point P1 (-58.5192, 1.6777)
  point P2 (-56.3799, 5.3832)
  point P3 (-51.1837, 2.3832)
  point P4 (-53.3231, -1.3223)
extrude "Extrusion6" cut sketch "Sketch15" against normal blind 2.3813
chamfer "Chamfer4" distance 0.24 angle 45 4 edges at (55.7082, 42.2906, 3.6512) (53.2082, 46.6207, 3.6512) (55.7082, 42.2906, 1.27) (53.2082, 46.6207, 1.27)
mirror "Mirror2" about plane through (68.1908, 39.37, 1.27) normal (-0.5, 0.8660254, 0) of "Hole4", "Hole5", "Hole6", "Extrusion5", "Extrusion6", "Chamfer4"
pattern_circular "Circular Pattern3" count 6 over 360 about axis through (0, 0, 1.27) along (0, 0, 1) of "Hole4", "Hole5", "Hole6", "Extrusion5", "Extrusion6", "Chamfer4", "Mirror2"
sketch "Sketch16" plane through (-0.3933, 42.4252, 8.89) normal (0, 0, 1) x (1, 0, 0)
  circle A0 centre (0.3933, -42.4252) radius 4.7625 projected
  circle A1 centre (15.8933, -57.9252) radius 5.175 projected
  circle A2 centre (-15.1067, -57.9252) radius 5.175 projected
  circle A3 centre (-40.4584, -66.0109) radius 15.605 projected
  arc A4 (58.5038, 14.4044) -> (20.5539, 36.3148) centre (0.3933, -42.4252) ccw projected
  line L0 (20.5539, 36.3148) -> (-19.7673, 36.3148) projected
  arc A5 (-19.7673, 36.3148) -> (-57.7172, 14.4044) centre (0.3933, -42.4252) ccw projected
  line L1 (-57.7172, 14.4044) -> (-77.8779, -20.5148) projected
  arc A6 (-77.8779, -20.5148) -> (-77.8779, -64.3356) centre (0.3933, -42.4252) ccw projected
  line L2 (-77.8779, -64.3356) -> (-57.7172, -99.2548) projected
  arc A7 (-57.7172, -99.2548) -> (-19.7673, -121.1652) centre (0.3933, -42.4252) ccw projected
  line L3 (-19.7673, -121.1652) -> (20.5539, -121.1652) projected
  arc A8 (20.5539, -121.1652) -> (58.5038, -99.2548) centre (0.3933, -42.4252) ccw projected
  line L4 (58.5038, -99.2548) -> (78.6644, -64.3356) projected
  arc A9 (78.6644, -64.3356) -> (78.6644, -20.5148) centre (0.3933, -42.4252) ccw projected
  line L5 (78.6644, -20.5148) -> (58.5038, 14.4044) projected
  circle A10 centre (0.3933, 4.7462) radius 15.605 projected
  circle A11 centre (41.2449, -66.0109) radius 15.605 projected
  circle A12 centre (-15.1067, -26.9252) radius 5.175 projected
  circle A13 centre (15.8933, -26.9252) radius 5.175 projected
  line L6 (-18.6567, -121.1652) -> (19.4433, -121.1652)
  line L7 (19.4433, -121.1652) -> (19.4433, -70.3652)
  line L8 (19.4433, -70.3652) -> (9.9183, -70.3652)
  line L9 (-18.6567, -70.3652) -> (-18.6567, -121.1652)
  line L10 (-18.6567, -121.1652) -> (19.4433, -70.3652) construction
  line L11 (19.4433, -121.1652) -> (-18.6567, -70.3652) construction
  line L12 (0.3933, -73.5402) -> (0.3933, -67.1902) construction
  line L13 (6.7433, -67.1902) -> (6.7433, -67.1902)
  line L14 (-5.9567, -67.1902) -> (-5.9567, -67.1902)
  arc A14 (-5.9567, -73.5402) -> (6.7433, -73.5402) centre (0.3933, -73.5402) ccw
  arc A15 (6.7433, -67.1902) -> (-5.9567, -67.1902) centre (0.3933, -67.1902) ccw
  line L15 (-9.1317, -70.3652) -> (-18.6567, -70.3652)
  arc A16 (-9.1317, -70.3652) -> (-5.9567, -67.1902) centre (-9.1317, -67.1902) ccw
  arc A17 (6.7433, -67.1902) -> (9.9183, -70.3652) centre (9.9183, -67.1902) ccw
  point P0 (0.3933, -95.7652)
  point P1 (0.3933, -95.7652)
  point P2 (0.3933, -121.1652)
  point P3 (0.3933, -70.3652)
  point P4 (0.3933, -70.3652)
  point P5 (0.3933, -121.1652)
  point P6 (6.7433, -67.1902)
  dimension "d95" = 38.1
  dimension "d96" = 50.8
  dimension "d97" = 3.175
  dimension "d98" = 12.7
  dimension "d99" = 3.175
  dimension "d100" = 19.05
  constraints: 22 end point, 8 point on circle, 8 tangent, 7 midpoint, 4 centre point, 4 parallel, 4 point on line, 3 perpendicular, 2 vertical alignment, 1 collinear, 1 equal radius, 1 horizontal
  measures "d95" distance of L6.start L6.end
  measures "d96" distance of L7.end L6.end
  measures "d97" distance of point (0.393, -70.365) L12.end
  measures "d98" diameter of A15
  measures "d99" radius of A16
  measures "d100" distance of L7.end point (0.393, -70.365)
sketch "Sketch17" plane through (-0.3933, 42.4252, 8.89) normal (0, 0, 1) x (1, 0, 0)
  line L0 (14.3707, -121.1652) -> (20.5539, -121.1652) projected
  line L1 (-19.7673, -70.3652) -> (20.5539, -70.3652)
  line L2 (20.5539, -70.3652) -> (20.5539, -121.1652)
  line L3 (20.5539, -121.1652) -> (-19.7673, -121.1652)
  line L4 (-19.7673, -121.1652) -> (-19.7673, -70.3652)
  line L5 (-19.7673, -70.3652) -> (20.5539, -121.1652) construction
  line L6 (20.5539, -70.3652) -> (-19.7673, -121.1652) construction
  point P0 (0.3933, -42.4252)
  point P1 (-18.6567, -70.3652)
  point P2 (19.4433, -70.3652)
  point P3 (0.3933, -95.7652)
  constraints: 12 end point, 2 midpoint, 2 parallel, 1 horizontal, 1 perpendicular
extrude "Extrusion7" add sketch "Sketch17" along normal blind 2
extrude "Extrusion8" cut sketch "Sketch16" along normal blind 1.2 contours L3 L9 L15 A16 A15 A17 L8 L7
sketch "Sketch18" plane through (-0.3933, 42.4252, 10.89) normal (0, 0, 1) x (1, 0, 0)
  line L0 (-18.6567, -70.3652) -> (-18.6567, -121.1652) projected
  line L1 (19.4433, -121.1652) -> (19.4433, -70.3652) projected
  line L2 (19.4433, -70.3652) -> (20.5539, -70.3652) construction
  line L3 (-18.6567, -121.1652) -> (19.4433, -70.3652) construction
  line L4 (19.4433, -121.1652) -> (19.4433, -70.3652) construction
  line L5 (-18.6567, -70.3652) -> (19.4433, -121.1652) construction
  line L6 (19.4433, -70.3652) -> (-18.6567, -70.3652) projected
  line L7 (-17.8567, -121.1652) -> (18.6433, -121.1652)
  line L8 (18.6433, -121.1652) -> (18.6433, -70.3652)
  line L9 (18.6433, -70.3652) -> (-17.8567, -70.3652)
  line L10 (-17.8567, -70.3652) -> (-17.8567, -121.1652)
  line L11 (-17.8567, -121.1652) -> (18.6433, -70.3652) construction
  line L12 (18.6433, -121.1652) -> (-17.8567, -70.3652) construction
  point P0 (0.3933, -42.4252)
  point P1 (0.3933, -95.7652)
  dimension "d105" = 0.8
  constraints: 16 end point, 3 midpoint, 2 parallel, 1 horizontal, 1 perpendicular, 1 point on line
  measures "d105" distance between parallel lines of L1 L8
extrude "Extrusion9" cut sketch "Sketch18" against normal up to surface (0.8 mm away)
chamfer "Chamfer5" distance 0.8 angle 45 6 edges at (-18.25, -53.34, 10.09) (-20.1606, -53.34, 10.89) (18.25, -53.34, 10.09) (20.1606, -53.34, 10.89) (20.1606, -53.34, 8.89) (-20.1606, -53.34, 8.89)
sketch "Sketch19" plane through (-20.9606, -27.94, 8.89) normal (0, 1, 0) x (1, 0, 0)
  line L0 (40.0106, 0) -> (1.9106, 0) projected
  line L1 (0.8, -1.2) -> (1.6, -2) projected
  line L2 (1.6, -2) -> (2.7106, -2) projected
  line L3 (0.8, -0.8) -> (0.8, -1.2) projected
  line L4 (1.6, -2) -> (0.8, -1.2)
  line L5 (0.8, -1.2) -> (0.8, 0)
  line L6 (0.8, 7.62) -> (0.8, -0.8) projected
  line L7 (0.8, 0) -> (5.88, 0)
  line L8 (5.88, 0) -> (5.88, -2)
  line L9 (5.88, -2) -> (1.6, -2)
  line L10 (1.9106, 0) -> (1.9106, -1.2) construction
  line L11 (1.9106, 0) -> (40.0106, 0) construction
  line L12 (20.9606, 0) -> (20.9606, 7.62) construction
  line L13 (12.3968, 7.62) -> (29.5244, 7.62) construction
  line L14 (41.1212, -1.2) -> (40.3212, -2)
  line L15 (40.3212, -2) -> (39.2106, -2)
  line L16 (41.1212, -0.8) -> (41.1212, -1.2)
  line L17 (40.3212, -2) -> (41.1212, -1.2)
  line L18 (41.1212, -1.2) -> (41.1212, 0)
  line L19 (41.1212, 0) -> (36.0412, 0)
  line L20 (36.0412, 0) -> (36.0412, -2)
  line L21 (36.0412, -2) -> (40.3212, -2)
  line L22 (40.0106, 0) -> (40.0106, -1.2) construction
  point P0 (20.9606, 8.89)
  point P1 (39.2106, -2)
  point P2 (41.1212, -0.8)
  point P3 (36.0412, 0)
  point P4 (1.9106, 0)
  dimension "d111" = 5.08
  constraints: 32 end point, 8 symmetric about line, 2 midpoint, 2 point on line, 1 collinear, 1 perpendicular
  measures "d111" distance of L5.end L7.end
extrude "Extrusion10" add sketch "Sketch19" along normal blind 2.54
chamfer "Chamfer6" distance 0.8 angle 45 6 edges at (-20.1606, -26.67, 8.89) (-17.6206, -25.4, 8.89) (17.0653, -25.4, 8.89) (20.1606, -26.67, 8.89) (17.2206, -25.4, 10.89) (-17.2206, -25.4, 10.89)
hole "Hole7" at (0, -24.765, 8.89) direction (0, 0, -1) diameter 4 depth 5.7
ref_plane "Work Plane3" through (68.1908, 39.37, 1.27) normal (-0.5, 0.8660254, 0) x (0, 0, 1)
ref_plane "Work Plane4" through (0, 78.74, 1.27) normal (-1, 0, 0) x (0, 0, 1)
ref_plane "Work Plane5" through (-68.1908, 39.37, 1.27) normal (-0.5, -0.8660254, 0) x (0, 0, 1)
ref_plane "Work Plane6" through (-68.1908, -39.37, 1.27) normal (0.5, -0.8660254, 0) x (0, 0, 1)
ref_plane "Work Plane7" through (0, -78.74, 1.27) normal (1, 0, 0) x (0, 0, 1)
ref_plane "Work Plane8" through (68.1908, -39.37, 1.27) normal (0.5, 0.8660254, 0) x (0, 0, 1)
body "Solid1"
